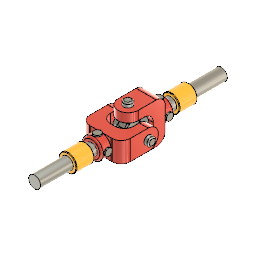
UNIV JOINT ASSEMN v0 (Autodesk Fusion 360 design; units mm, degrees)
Autodesk Fusion 360 part; units mm, degrees
note: some values were not read from the file. Chosen so that the rebuilt part matches the saved one: which face or edge a step refers to; which bodies a step acts on.
sketch "Sketch1" plane through (0, 0, 0) normal (0, 0, 1) x (1, 0, 0)
  line L0 (16.9775, 0) -> (51.0225, 0)
  line L1 (68, 31) -> (68, 78)
  line L2 (0, 78) -> (0, 31)
  line L3 (53, 51) -> (53, 78)
  line L4 (15, 51) -> (15, 78)
  line L5 (30, 36) -> (38, 36)
  arc A0 (38, 36) -> (53, 51) centre (38, 51) ccw
  arc A1 (15, 51) -> (30, 36) centre (30, 51) ccw
  line L6 (16.9775, 0) -> (16.9775, 16)
  line L7 (16.9775, 16) -> (15, 16)
  line L8 (51.0225, 0) -> (51.0225, 16)
  line L9 (51.0225, 16) -> (53, 16)
  line L10 (68, 78) -> (53, 78)
  line L11 (15, 78) -> (0, 78)
  arc A2 (53, 16) -> (68, 31) centre (53, 31) ccw
  arc A3 (0, 31) -> (15, 16) centre (15, 31) ccw
  point P0 (53, 36)
  dimension "d2" = 78
  dimension "d5" = 42
  dimension "d6" = 15
  dimension "d7" = 15
  dimension "d8" = 16
  dimension "d9" = 15
  dimension "d10" = 15
  constraint horizontal L0
  constraint vertical L1
  constraint horizontal L10
  constraint vertical L2
  constraint vertical L3
  constraint coincident P0 L3
  constraint coincident P0 L5
  constraint tangent L3 A0
  constraint tangent L5 A0
  constraint tangent L4 A1
  constraint tangent L5 A1
  constraint perpendicular L0 L6
  constraint perpendicular L2 L7
  constraint collinear L10 L11
  constraint tangent L9 A2
  constraint tangent L1 A2
  constraint tangent L7 A3
  constraint tangent L2 A3
  measures "d2" distance of origin L2.start
  measures "d5" distance of P0 L3.end
  measures "d6" radius of A0
  measures "d7" radius of A1
  measures "d8" distance of L0.start L6.end
  measures "d9" radius of A2
  measures "d10" radius of A3
extrude "Extrude1" add sketch "Sketch1" along normal blind 34 makes body 1
fillet "Fillet1" radius 3 2 edges at (16.9775, 0, 17) (51.0225, 0, 17) on bodies 1
sketch "Sketch2" plane through (0, 0, 0) normal (0, -1, 0) x (1, 0, 0)
  line L0 (48.0225, 0) -> (48.0225, 34)
  line L1 (48.0225, 34) -> (19.9775, 34)
  line L2 (19.9775, 34) -> (19.9775, 0)
  line L3 (19.9775, 0) -> (48.0225, 0)
  circle A0 centre (34, 17) radius 9.5
  dimension "d16" = 19
  measures "d16" diameter of A0
extrude "Extrude2" cut sketch "Sketch2" against normal blind 95 contours A0 bodies 1
fillet "Fillet2" radius 2 4 edges at (68, 78, 17) (53, 78, 17) (15, 78, 17) (0, 78, 17) on bodies 1
sketch "Sketch3" plane through (68, 0, 0) normal (1, 0, 0) x (0, 1, 0)
  line L0 (76, 0) -> (76, 34)
  line L1 (76, 34) -> (31, 34)
  line L2 (31, 34) -> (31, 0)
  line L3 (31, 0) -> (76, 0)
  circle A0 centre (61.5, 17) radius 6
  dimension "d23" = 12
  measures "d23" diameter of A0
delete_face "DeleteFace1" 1 faces at (66.3785, 77.9639, 11.3333) on bodies 1
delete_face "DeleteFace2" 3 faces at (53.5525, 77.3802, 11.3333) (14.4475, 77.3802, 11.3333) (0.8399, 77.6292, 11.3333) on bodies 1
extrude "Extrude3" cut sketch "Sketch3" against normal blind 100 contours A0 bodies 1
fillet "Fillet3" radius 17 2 edges at (60.5, 78, 34) (60.5, 78, 0) on bodies 1
fillet "Fillet4" radius 17 2 edges at (7.5, 78, 34) (7.5, 78, 0) on bodies 1
delete_face "DeleteFace3" 2 faces at (48.1653, 0.0034, 11.3333) (19.8347, 0.0034, 11.3333) on bodies 1
sketch "Sketch4" plane through (0, 0, 0) normal (0, -1, 0) x (1, 0, 0)
  line L0 (16.9775, 34) -> (16.9775, 0)
  line L1 (16.9775, 0) -> (51.0225, 0)
  line L2 (51.0225, 0) -> (51.0225, 34)
  line L3 (51.0225, 34) -> (16.9775, 34)
  circle A0 centre (34, 17) radius 9.5
  circle A1 centre (34, 17) radius 17
  line L4 (15, 40) -> (55, 40)
  line L5 (55, 40) -> (55, -5)
  line L6 (55, -5) -> (15, -5)
  line L7 (15, -5) -> (15, 40)
  dimension "d30" = 34
  constraint concentric A0 A1
  constraint horizontal L4
  constraint vertical L5
  constraint horizontal L6
  constraint vertical L7
  measures "d30" diameter of A1
extrude "Extrude4" cut sketch "Sketch4" against normal blind 15.9 contours L0 L1 L3 A1 | L1 L2 L3 A1 | L4 L5 L6 L7 bodies 1
fillet "Fillet5" radius 3 1 edges at (18.1504, 0, 10.8525) on bodies 1
sketch "Sketch5" plane through (0, 0, 0) normal (0, -1, 0) x (1, 0, 0)
  circle A0 centre (34, 17) radius 9.5
  circle A1 centre (34, 17) radius 14
  circle A2 centre (34, 17) radius 15
  circle A3 centre (34, 17) radius 10
  dimension "d35" = 30
  dimension "d36" = 20
  constraint concentric A0 A2
  constraint concentric A2 A3
  measures "d35" diameter of A2
  measures "d36" diameter of A3
extrude "Extrude5" add sketch "Sketch5" along normal blind 30 separate body contours A1 | A2 makes body 2
move_body "Move1" bodies 2 to x (1, 0, 0) y (0, 1, 0) z (0, 0, 1) at (0, -10, 0)
sketch "Sketch6" plane through (0, -40, 0) normal (0, -1, 0) x (1, 0, 0)
  circle A0 centre (34, 17) radius 10
  circle A1 centre (34, 17) radius 15
  circle A2 centre (34, 17) radius 8.5
  dimension "d39" = 17
  constraint concentric A0 A2
  measures "d39" diameter of A2
extrude "Extrude6" add sketch "Sketch6" against normal blind 7 separate body contours A2 makes body 3
sketch "Sketch7" plane through (0, -33, 0) normal (0, 1, 0) x (-1, 0, 0)
  circle A0 centre (-34, 17) radius 8.5
  circle A1 centre (-34, 17) radius 7.5
  dimension "d42" = 15
  constraint concentric A0 A1
  measures "d42" diameter of A1
extrude "Extrude7" add sketch "Sketch7" along normal blind 6 separate body contours A1 makes body 4
copy_body "CopyPasteBodies1" bodies 3 makes body 5
move_body "Move2" bodies 5 to x (1, 0, 0) y (0, 1, 0) z (0, 0, 1) at (0, 13, 0)
combine "Combine1" operation add target body 5 tool bodies 4 3
sketch "Sketch8" plane through (0, -40, 0) normal (0, -1, 0) x (1, 0, 0)
  circle A0 centre (34, 17) radius 8.5
  circle A1 centre (34, 17) radius 12.5
  dimension "d48" = 25
  constraint concentric A0 A1
  measures "d48" diameter of A1
extrude "Extrude8" add sketch "Sketch8" along normal blind 10 contours A0 | A1 bodies 5
sketch "Sketch9" plane through (0, -50, 0) normal (0, -1, 0) x (1, 0, 0)
  circle A0 centre (34, 17) radius 12.5
  circle A1 centre (34, 17) radius 10
  dimension "d51" = 20
  constraint concentric A0 A1
  measures "d51" diameter of A1
extrude "Extrude9" add sketch "Sketch9" along normal blind 100 contours A1 bodies 5
move_body "Move3" bodies 5 to x (1, 0, 0) y (0, 1, 0) z (0, 0, 1) at (0, 55, 0)
chamfer "Chamfer1" distance 1 angle 45 2 edges at (20.0151, -10, 11.5758) (20.0151, -40, 11.5758) on bodies 2
ref_plane "WorkPlane1" through (0, 0, 35) normal (0, 0, 1) x (1, 0, 0)
sketch "Sketch10" plane through (0, 0, 35) normal (0, 0, 1) x (1, 0, 0)
  circle A0 centre (34, 10) radius 3
  dimension "d59" = 6
  measures "d59" diameter of A0
extrude "Extrude10" cut sketch "Sketch10" against normal blind 12 bodies 1 5
pattern_circular "C-Pattern1" count 4 over 360 about axis through (34, 3, 17) along (0, 1, 0) of 1 faces at (36.4654, 11.7094, 28.7265) on bodies 1
move_body "Move4" bodies 1 2 5 to x (1, 0, 0) y (0, 1, 0) z (0, 0, 1) at (0, -100, 0)
sketch "Sketch11" plane through (0, 0, 0) normal (0, 0, 1) x (1, 0, 0)
  circle A0 centre (30, 30) radius 3
  dimension "d67" = 6
  measures "d67" diameter of A0
extrude "Extrude11" add sketch "Sketch11" along normal blind 10 separate body makes body 6
sketch "Sketch12" plane through (0, 0, 10) normal (0, 0, 1) x (-1, 0, 0)
  circle A0 centre (-30, -30) radius 3
  circle A1 centre (-30, -30) radius 6
  dimension "d70" = 12
  constraint concentric A0 A1
  measures "d70" diameter of A1
extrude "Extrude12" add sketch "Sketch12" along normal blind 2 contours A0 | A1 bodies 6
move_body "Move5" bodies 6 to x (1, 0, 0) y (0, 1, 0) z (0, 0, 1) at (4, -120, 34)
pattern_circular "C-Pattern2" count 4 over 360 about axis through (34, -97, 17) along (0, 1, 0) of bodies 6 makes body 7 at (57.6667, -91.5643, 19.5599) makes body 8 at (36.5599, -91.5643, -6.6667) makes body 9 at (10.3333, -91.0261, 19.8191)
move_body "Move6" bodies 6 to x (1, 0, 0) y (0, 1, 0) z (0, 0, 1) at (0, 0, -10)
move_body "Move7" bodies 7 to x (1, 0, 0) y (0, 1, 0) z (0, 0, 1) at (-10, 0, 0)
move_body "Move8" bodies 9 to x (1, 0, 0) y (0, 1, 0) z (0, 0, 1) at (10, 0, 0)
move_body "Move9" bodies 8 to x (1, 0, 0) y (0, 1, 0) z (0, 0, 1) at (0, 0, 10)
mirror "Mirror1" about plane through (0, 0, 0) normal (0, 1, 0) of bodies 6 1 2 7 5 8 9 makes body 10 at (5.0509, 53.0438, 34) makes body 11 at (48.9814, 129.6667, 16.2523) makes body 12 at (46.4379, 88.3333, 15.7554) makes body 13 at (34.445, 91.9499, 36) makes body 14 at (53, 91.9499, 16.555) makes body 15 at (37.9777, 90.2981, -2) makes body 16 at (15, 88.0501, 16.555)
move_body "Move10" bodies 12 16 15 10 11 14 13 to x (0, 0, 1) y (0, 1, 0) z (-1, 0, 0) at (51, 0, -17)
sketch "Sketch13" plane through (0, 0, 0) normal (1, 0, 0) x (0, 1, 0)
  circle A0 centre (0, 150) radius 6
  line L0 (7.7, 137.3) -> (-7.7, 137.3)
  line L1 (-12.7, 142.3) -> (-12.7, 157.7)
  line L2 (-7.7, 162.7) -> (7.6, 162.7)
  line L3 (12.7, 157.7) -> (12.7, 142.3)
  line L4 (12.7, 137.3) -> (-12.7, 162.7) construction
  line L5 (-12.7, 137.3) -> (12.7, 162.7) construction
  line L6 (-7.7, 162.7) -> (-12.7, 157.7)
  line L7 (7.6, 162.7) -> (12.7, 157.7)
  line L8 (12.7, 142.3) -> (7.7, 137.3)
  line L9 (-7.7, 137.3) -> (-12.7, 142.3)
  point P0 (0, 150)
  dimension "d93" = 12
  dimension "d94" = 25.4
  dimension "d95" = 25.4
  dimension "d96" = 5
  dimension "d97" = 5
  dimension "d98" = 5.1
  dimension "d99" = 5
  dimension "d100" = 5
  dimension "d101" = 5
  dimension "d102" = 5
  dimension "d103" = 5
  constraint horizontal L0
  constraint perpendicular L0 L1
  constraint parallel L0 L2
  constraint parallel L1 L3
  constraint coincident L4 P0
  constraint coincident L5 P0
  constraint coincident P0 A0.centre
  constraint coincident L4.end L2
  constraint coincident L4.end L1
  constraint coincident L5.end L2
  constraint coincident L5.end L3
  constraint coincident L4.start L3
  constraint coincident L4.start L0
  constraint coincident L5.start L0
  constraint coincident L5.start L1
  measures "d93" diameter of A0
  measures "d94" distance of L4.end L5.end
  measures "d95" distance of L5.start L4.end
  measures "d96" distance of L4.end L2.start
  measures "d97" distance of L4.end L1.end
  measures "d98" distance of L5.end L2.end
  measures "d99" distance of L5.end L3.start
  measures "d100" distance of L4.start L3.end
  measures "d101" distance of L4.start L0.start
  measures "d102" distance of L5.start L0.end
  measures "d103" distance of L5.start L1.start
extrude "Extrude13" add sketch "Sketch13" along normal blind 15 separate body makes body 17
sketch "Sketch14" plane through (0, -12.7, 0) normal (0, -1, 0) x (1, 0, 0)
  line L0 (0, 157.7) -> (0, 142.3)
  line L1 (0, 142.3) -> (15, 142.3)
  line L2 (15, 142.3) -> (15, 157.7)
  line L3 (15, 157.7) -> (0, 157.7)
  circle A0 centre (7.5, 150) radius 6
  dimension "d106" = 12
  measures "d106" diameter of A0
extrude "Extrude14" cut sketch "Sketch14" against normal blind 45 contours A0 bodies 17
sketch "Sketch15" plane through (0, 0, 162.7) normal (0, 0, 1) x (-1, 0, 0)
  line L0 (0, -7.6) -> (0, 7.7)
  line L1 (0, 7.7) -> (-15, 7.7)
  line L2 (-15, 7.7) -> (-15, -7.6)
  line L3 (-15, -7.6) -> (0, -7.6)
  circle A0 centre (-7.5, 0) radius 6
  dimension "d109" = 7.5
  dimension "d110" = 12
  measures "d109" distance of origin A0.centre
  measures "d110" diameter of A0
extrude "Extrude15" cut sketch "Sketch15" against normal blind 35 contours A0 bodies 17
chamfer "Chamfer2" distance 2 angle 45 8 edges at (15, 10.15, 160.2) (15, -10.2, 160.2) (15, -10.2, 139.8) (15, 10.2, 139.8) (0, -10.2, 160.2) (0, 10.15, 160.2) (0, 10.2, 139.8) (0, -10.2, 139.8) on bodies 17
move_body "Move11" bodies 17 to x (1, 0, 0) y (0, 1, 0) z (0, 0, 1) at (26.8, 0, 0)
move_body "Move12" bodies 17 to x (1, 0, 0) y (0, 1, 0) z (0, 0, 1) at (0, 0, -130)
move_body "Move13" bodies 12 10 14 13 16 15 11 to x (1, 0, 0) y (0, 1, 0) z (0, 0, 1) at (0, -39, 0)
move_body "Move14" bodies 9 7 5 2 8 6 1 to x (1, 0, 0) y (0, 1, 0) z (0, 0, 1) at (0, 38.5, 0)
move_body "Move15" bodies 17 to x (1, 0, 0) y (0, 1, 0) z (0, 0, 1) at (0, 0, -3)
sketch "Sketch16" plane through (0, 0, 51) normal (0, 0, 1) x (-1, 0, 0)
  circle A0 centre (-34, 0.5) radius 6
  arc A1 (-17, 0) -> (-51, 0) centre (-34, 0) ccw
  line L0 (-51, 0) -> (-51, -30)
  line L1 (-51, -30) -> (-17, -30)
  line L2 (-17, -30) -> (-17, 0)
  circle A2 centre (-34, 0.5) radius 6
  dimension "d129" = 12
  constraint concentric A0 A2
  measures "d129" diameter of A2
extrude "Extrude16" add sketch "Sketch16" along normal blind 33 separate body contours A0 A2 makes body 18
sketch "Sketch17" plane through (0, 0, 84) normal (0, 0, 1) x (-1, 0, 0)
  circle A0 centre (-34, 0.5) radius 6
  circle A1 centre (-34, 0.5) radius 7
  dimension "d132" = 14
  constraint concentric A0 A1
  measures "d132" diameter of A1
extrude "Extrude17" add sketch "Sketch17" along normal blind 7 contours A0 | A1 bodies 18
move_body "Move16" bodies 18 to x (1, 0, 0) y (0, 1, 0) z (0, 0, 1) at (0, 0, -33)
fillet "Fillet6" radius 2 1 edges at (40.5263, 2.0313, 58) on bodies 18
pattern_circular "C-Pattern3" count 4 over 360 about axis through (34, -56.5, 17) along (0, -1, 0) of bodies 18 makes body 19 at (11, 0.0974, 11.0298) makes body 20 at (39.9702, 0.0974, -6) makes body 21 at (57, 0.0974, 22.9702)
equation "d103 = d102"
named bodies: "Body3", "Body4", "Body4 (1)", "Body4 (2)", "Body4 (3)", "Body3 (1)", "Body4 (4)", "Body4 (1) (1)", "Body4 (2) (1)", "Body4 (3) (1)"
